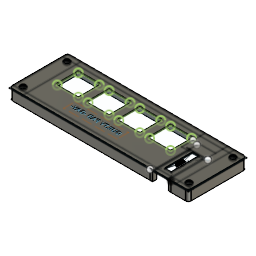
case-top (Autodesk Fusion 360 design; units mm, degrees)
part number: 2025-11-22-15-29-30-254
Autodesk Fusion 360 part; units mm, degrees
sketch "layout" plane through (0, 0, 0) normal (0, 0, 1) x (1, 0, 0)
  line L0 (0.025, -13.525) -> (0.025, -0.525)
  line L1 (14.025, -13.525) -> (14.025, -0.525)
  line L2 (0.525, -14.025) -> (13.525, -14.025)
  line L3 (0.525, -0.025) -> (13.525, -0.025)
  arc A0 (0.025, -13.525) -> (0.525, -14.025) centre (0.525, -13.525) ccw
  arc A1 (0.525, -0.025) -> (0.025, -0.525) centre (0.525, -0.525) ccw
  arc A2 (13.525, -14.025) -> (14.025, -13.525) centre (13.525, -13.525) ccw
  arc A3 (14.025, -0.525) -> (13.525, -0.025) centre (13.525, -0.525) ccw
  line L4 (19.075, -13.525) -> (19.075, -0.525)
  line L5 (33.075, -13.525) -> (33.075, -0.525)
  line L6 (19.575, -14.025) -> (32.575, -14.025)
  line L7 (19.575, -0.025) -> (32.575, -0.025)
  arc A4 (19.075, -13.525) -> (19.575, -14.025) centre (19.575, -13.525) ccw
  arc A5 (19.575, -0.025) -> (19.075, -0.525) centre (19.575, -0.525) ccw
  arc A6 (32.575, -14.025) -> (33.075, -13.525) centre (32.575, -13.525) ccw
  arc A7 (33.075, -0.525) -> (32.575, -0.025) centre (32.575, -0.525) ccw
  line L8 (38.125, -13.525) -> (38.125, -0.525)
  line L9 (52.125, -13.525) -> (52.125, -0.525)
  line L10 (38.625, -14.025) -> (51.625, -14.025)
  line L11 (38.625, -0.025) -> (51.625, -0.025)
  arc A8 (38.125, -13.525) -> (38.625, -14.025) centre (38.625, -13.525) ccw
  arc A9 (38.625, -0.025) -> (38.125, -0.525) centre (38.625, -0.525) ccw
  arc A10 (51.625, -14.025) -> (52.125, -13.525) centre (51.625, -13.525) ccw
  arc A11 (52.125, -0.525) -> (51.625, -0.025) centre (51.625, -0.525) ccw
  line L12 (57.175, -13.525) -> (57.175, -0.525)
  line L13 (71.175, -13.525) -> (71.175, -0.525)
  line L14 (57.675, -14.025) -> (70.675, -14.025)
  line L15 (57.675, -0.025) -> (70.675, -0.025)
  arc A12 (57.175, -13.525) -> (57.675, -14.025) centre (57.675, -13.525) ccw
  arc A13 (57.675, -0.025) -> (57.175, -0.525) centre (57.675, -0.525) ccw
  arc A14 (70.675, -14.025) -> (71.175, -13.525) centre (70.675, -13.525) ccw
  arc A15 (71.175, -0.525) -> (70.675, -0.025) centre (70.675, -0.525) ccw
  line L16 (-12.6365, 6.026) -> (98.1475, 6.026)
  line L17 (98.1475, 6.026) -> (98.1475, -29.974)
  line L18 (98.1475, -29.974) -> (-12.6365, -29.974)
  line L19 (-12.6365, -29.974) -> (-12.6365, 6.026)
  line L20 (85.8249, -7.074) -> (75.9249, -7.074)
  line L21 (75.9249, -7.074) -> (75.9249, -29.974)
  line L22 (75.9249, -29.974) -> (85.8249, -29.974)
  line L23 (85.8249, -29.974) -> (85.8249, -7.074)
  line L24 (85.8249, -7.074) -> (75.9249, -29.974) construction
  line L25 (75.9249, -7.074) -> (85.8249, -29.974) construction
  line L26 (76.5749, -29.974) -> (76.5749, -7.074)
  line L27 (85.1749, -29.974) -> (85.1749, -7.074)
  line L28 (82.875, -25.314) -> (78.875, -25.314)
  line L29 (78.875, -25.314) -> (78.875, -8.074)
  line L30 (78.875, -8.074) -> (82.875, -8.074)
  line L31 (82.875, -8.074) -> (82.875, -25.314)
  line L32 (82.875, -25.314) -> (78.875, -8.074) construction
  line L33 (78.875, -25.314) -> (82.875, -8.074) construction
  line L34 (-12.6365, 3.326) -> (98.1475, 3.326)
  line L35 (86.1475, 3.326) -> (86.1475, 6.026)
  line L36 (72.1475, 3.326) -> (72.1475, 6.026)
  circle A16 centre (94.1475, -25.574) radius 1.7
  circle A17 centre (94.1475, 1.626) radius 1.7
  circle A18 centre (-8.6365, -25.574) radius 1.7
  circle A19 centre (-8.6365, 1.626) radius 1.7
  line L37 (90.1475, -29.974) -> (90.1475, 6.026)
  line L38 (-4.6365, -29.974) -> (-4.6365, 6.026)
  line L39 (98.1475, -27.274) -> (-12.6365, -27.274)
  line L40 (75.9249, -29.974) -> (74.4249, -29.974)
  line L41 (75.9249, -2.474) -> (75.9249, -29.974)
  line L42 (85.8249, -29.974) -> (87.3249, -29.974)
  line L43 (75.9249, -29.974) -> (74.4249, -29.974)
  line L44 (87.3249, -29.974) -> (85.8249, -29.974)
  line L45 (74.4249, -7.074) -> (75.9249, -7.074)
  line L46 (85.8249, -7.074) -> (87.3249, -7.074)
  line L47 (74.4249, -7.074) -> (87.3249, -7.074)
  line L48 (86.1475, 3.326) -> (86.1475, -8.174)
  line L49 (86.1475, -8.174) -> (72.1475, -8.174)
  line L50 (72.1475, -8.174) -> (72.1475, 3.326)
  line L51 (86.1475, -1.174) -> (72.1475, -1.174)
  point P0 (80.8749, -18.524)
  point P1 (80.875, -16.694)
  dimension "d1" = 110.784
  dimension "d2" = 36
  dimension "d3" = 12.6615
  dimension "d4" = 15.949
  dimension "d10" = 9.9
  dimension "d11" = 22.9
  dimension "d14" = 0.65
  dimension "d15" = 0.65
  dimension "d16" = 0.0001
  dimension "d17" = 4
  dimension "d18" = 9.62
  dimension "d19" = 17.24
  dimension "d20" = 9.7
  dimension "d22" = 2.7
  dimension "d23" = 12
  dimension "d24" = 14
  dimension "d25" = 3.4
  dimension "d26" = 4.4
  dimension "d27" = 4
  dimension "d28" = 3.4
  dimension "d29" = 4
  dimension "d30" = 4.4
  dimension "d31" = 3.4
  dimension "d32" = 4.4
  dimension "d33" = 4
  dimension "d34" = 3.4
  dimension "d35" = 4.4
  dimension "d36" = 4
  dimension "d37" = 8
  dimension "d38" = 8
  dimension "d39" = 2.7
  dimension "d49" = 1.5
  dimension "d75" = 8.75
  dimension "d83" = 11.5
  dimension "d84" = 4.5
  constraint horizontal L16
  constraint vertical L17
  constraint horizontal L18
  constraint vertical L19
  constraint horizontal L20
  constraint perpendicular L20 L21
  constraint parallel L20 L22
  constraint parallel L21 L23
  constraint coincident L24 P0
  constraint coincident L25 P0
  constraint coincident L22 L26.start
  constraint coincident L20 L26.end
  constraint perpendicular L20 L26
  constraint coincident L22 L27.start
  constraint coincident L20 L27.end
  constraint perpendicular L20 L27
  constraint horizontal L28
  constraint perpendicular L28 L29
  constraint parallel L28 L30
  constraint parallel L29 L31
  constraint coincident L32 P1
  constraint coincident L33 P1
  constraint coincident L19 L34.start
  constraint coincident L17 L34.end
  constraint perpendicular L17 L34
  constraint coincident L34 L35.start
  constraint coincident L16 L35.end
  constraint perpendicular L16 L35
  constraint coincident L34 L36.start
  constraint coincident L16 L36.end
  constraint perpendicular L16 L36
  constraint coincident L18 L37.start
  constraint coincident L16 L37.end
  constraint perpendicular L16 L37
  constraint coincident L18 L38.start
  constraint coincident L16 L38.end
  constraint perpendicular L16 L38
  constraint coincident L17 L39.start
  constraint coincident L19 L39.end
  constraint perpendicular L19 L39
  constraint coincident L18 L40.end
  constraint coincident L18 L42.end
  constraint horizontal L40
  constraint vertical L41
  constraint horizontal L42
  constraint perpendicular L21 L45
  constraint horizontal L47
  constraint perpendicular L34 L48
  constraint perpendicular L36 L49
  constraint perpendicular L34 L50
  constraint coincident L48 L51.start
  constraint perpendicular L48 L51
  measures "d1" distance of L16.start L16.end
  measures "d2" distance of L16 L18
  measures "d3" distance of L0 L19
  measures "d4" distance of L2 L18
  measures "d10" distance of L21 L23
  measures "d11" distance of L20 L22
  measures "d14" distance of L21 L26
  measures "d15" distance of L23 L27
  measures "d16" horizontal distance of P0 P1
  measures "d17" distance of L29 L31
  measures "d18" distance of L20 P1
  measures "d19" distance of L28 L30
  measures "d20" distance of L13 P1
  measures "d22" distance of L16 L34
  measures "d23" distance of L17 L35
  measures "d24" distance of L35 L36
  measures "d25" diameter of A16
  measures "d26" distance of L18 A16.centre
  measures "d27" distance of L17 A16.centre
  measures "d28" diameter of A17
  measures "d29" distance of L17 A17.centre
  measures "d30" distance of L16 A17.centre
  measures "d31" diameter of A18
  measures "d32" distance of L18 A18.centre
  measures "d33" distance of L19 A18.centre
  measures "d34" diameter of A19
  measures "d35" distance of L16 A19.centre
  measures "d36" distance of L19 A19.centre
  measures "d37" distance of L17 L37
  measures "d38" distance of L19 L38
  measures "d39" distance of L18 L39
  measures "d49" distance of L22.end L42.end
  measures "d75" distance of P0 L39
  measures "d83" distance of L35.start L48.end
  measures "d84" distance of L34 L51
extrude "Extrude1" add sketch "layout" along normal blind 0.6 contours L16 L19 L34 L38 | L16 L34 L36 L38 | L19 L34 L38 L39 | L16 L34 L35 L36 | L21 L34 L38 L39 L41 L49 L50 | L18 L19 L38 L39 | L16 L34 L35 L37 | L34 L48 L50 L51 | L18 L21 L38 L39 L40 L41 L43 | L16 L17 L34 L37 | L23 L34 L37 L39 L48 L49 | L20 L21 L41 L46 L47 L48 L49 L50 L51 | L18 L21 L22 L26 L39 L41 | L21 L26 L39 L41 L49 | L17 L34 L37 L39 | L20 L21 L26 L41 L47 L49 | L18 L22 L26 L27 L39 | L26 L27 L28 L29 L31 L39 L49 | L17 L18 L37 L39 | L18 L23 L37 L39 L42 L44 | L23 L46 L47 L48 L49 | L20 L26 L27 L29 L30 L31 L47 L49 | L18 L22 L23 L27 L39 | L23 L27 L39 L49 | L20 L23 L27 L47 L49 makes body 1
extrude "Extrude2" add sketch "layout" against normal blind 6 separate body contours L16 L19 L34 L38 | L16 L34 L36 L38 | L19 L34 L38 L39 | L18 L19 L38 L39 | L16 L34 L35 L37 | L18 L21 L38 L39 L40 L41 L43 | L16 L17 L34 L37 | L17 L34 L37 L39 | L17 L18 L37 L39 | L18 L23 L37 L39 L42 L44 makes body 2 at (-5.5544, -7.8261, 0) makes body 3 at (92.6881, 5.1118, 0)
sketch "daughterboard carrier overhang" plane through (0, 0, -2) normal (0, 0, -1) x (1, 0, 0)
  line L0 (75.9249, 1.274) -> (75.9249, 27.274)
  line L1 (75.9249, 1.274) -> (76.5749, 1.274)
  line L2 (76.5749, 1.274) -> (76.5749, 26.274)
  line L3 (76.5749, 26.274) -> (75.9249, 26.274)
  line L4 (75.9249, 26.274) -> (75.9249, 1.274)
  line L5 (75.9249, 27.274) -> (74.4249, 27.274)
  line L6 (74.4249, 27.274) -> (74.4249, 0.274)
  line L7 (74.4249, 0.274) -> (75.9249, 0.274)
  line L8 (75.9249, 0.274) -> (75.9249, 27.274)
  line L9 (85.1749, 0.274) -> (85.8249, 0.274)
  line L10 (85.8249, 0.274) -> (85.8249, 26.274)
  line L11 (85.8249, 26.274) -> (85.1749, 26.274)
  line L12 (85.1749, 26.274) -> (85.1749, 0.274)
  line L13 (85.8249, 0.274) -> (87.3249, 0.274)
  line L14 (87.3249, 0.274) -> (87.3249, 26.274)
  line L15 (87.3249, 26.274) -> (85.8249, 26.274)
  line L16 (85.8249, 26.274) -> (85.8249, 0.274)
  line L17 (85.8249, 27.274) -> (85.8249, 1.274)
  line L18 (85.8249, 1.274) -> (75.9249, 1.274)
  line L19 (75.9249, 27.274) -> (-4.6365, 27.274)
  line L20 (-4.6365, 27.274) -> (-4.6365, -3.326)
  line L21 (-4.6365, -3.326) -> (90.1475, -3.326)
  line L22 (90.1475, -3.326) -> (90.1475, 27.274)
  line L23 (90.1475, 27.274) -> (85.8249, 27.274)
  line L24 (75.9249, 26.274) -> (74.4249, 26.274)
  line L25 (76.5749, 26.274) -> (75.9249, 26.274)
  line L26 (75.9249, 26.274) -> (75.9249, 27.274)
  line L27 (75.9249, 27.274) -> (76.5749, 27.274)
  line L28 (76.5749, 27.274) -> (76.5749, 26.274)
  line L29 (85.1749, 26.274) -> (85.8249, 26.274)
  line L30 (85.8249, 26.274) -> (85.8249, 27.274)
  line L31 (85.8249, 27.274) -> (85.1749, 27.274)
  line L32 (85.1749, 27.274) -> (85.1749, 26.274)
  line L33 (85.8249, 26.274) -> (85.1749, 26.274)
  line L34 (85.1749, 26.274) -> (85.1749, 27.274)
  line L35 (85.1749, 27.274) -> (85.8249, 27.274)
  line L36 (85.8249, 27.274) -> (85.8249, 26.274)
  line L37 (87.3249, 26.274) -> (87.3249, 27.274)
  line L38 (85.8249, 27.274) -> (87.3249, 27.274)
  line L39 (87.3249, 27.274) -> (87.3249, 29.974)
  line L40 (87.3249, 29.974) -> (85.8249, 27.274)
  line L41 (74.4249, 27.274) -> (74.4249, 29.974)
  line L42 (74.4249, 29.974) -> (75.9249, 27.274)
  dimension "d52" = 0.65
  dimension "d60" = 0.65
  dimension "d61" = 26
  dimension "d62" = 8.6
  dimension "d63" = 1.5
  dimension "d64" = 26
  dimension "d76" = 26
  dimension "d77" = 2.7
  dimension "d78" = 1.5
  dimension "d79" = 2.7
  constraint horizontal L1
  constraint vertical L2
  constraint horizontal L3
  constraint vertical L4
  constraint coincident L0.start L1.start
  constraint horizontal L5
  constraint vertical L6
  constraint horizontal L7
  constraint vertical L8
  constraint coincident L0.end L5.start
  constraint horizontal L9
  constraint vertical L10
  constraint horizontal L11
  constraint vertical L12
  constraint horizontal L13
  constraint vertical L14
  constraint horizontal L15
  constraint vertical L16
  constraint coincident L6 L24.end
  constraint perpendicular L6 L24
  constraint horizontal L25
  constraint vertical L26
  constraint horizontal L27
  constraint vertical L28
  constraint horizontal L29
  constraint vertical L30
  constraint horizontal L31
  constraint vertical L32
  constraint coincident L17.start L23.end
  constraint horizontal L33
  constraint vertical L34
  constraint horizontal L35
  constraint vertical L36
  constraint coincident L23 L37.end
  constraint perpendicular L23 L37
  constraint perpendicular L23 L39
  constraint perpendicular L5 L41
  measures "d52" distance of L2 L4
  measures "d60" distance of L9.start L9.end
  measures "d61" distance of L9.start L11.end
  measures "d62" distance of L2 L12
  measures "d63" distance of L9.end L13.end
  measures "d64" distance of L9.end L10.end
  measures "d76" distance of L7 L24
  measures "d77" distance of L37.end L39.end
  measures "d78" distance of L6 L8
  measures "d79" distance of L5.end L41.end
fillet "Fillet1" radius 1.7 8 edges at (98.1475, -29.974, 0.3) (98.1475, 6.026, 0.3) (-12.6365, 6.026, 0.3) (-12.6365, -29.974, 0.3) (-12.6365, 6.026, -3) (-12.6365, -29.974, -3) (98.1475, -29.974, -3) (98.1475, 6.026, -3) on bodies 1 2 3
sketch "Sketch3" plane through (0, 0, 0) normal (0, 0, 1) x (1, 0, 0)
  line L0 (48, -24) -> (15, -24) construction
  line L1 (15, -24) -> (15, -17) construction
  line L2 (15, -17) -> (48, -17) construction
  line L3 (48, -17) -> (48, -24) construction
  dimension "d69" = 2.5
  text T0 "GUILTY PAD -GAY-" font "Arial" height 2.5 align centre middle in box 33 x 7 at (48, -24) x (-1, 0) y (0, 1) spacing 1 kerned
extrude "Extrude6" cut sketch "Sketch3" along normal blind 0.2 text T0 bodies 1
equation "d70 = 'GUILTY PAD -GAY-'"
